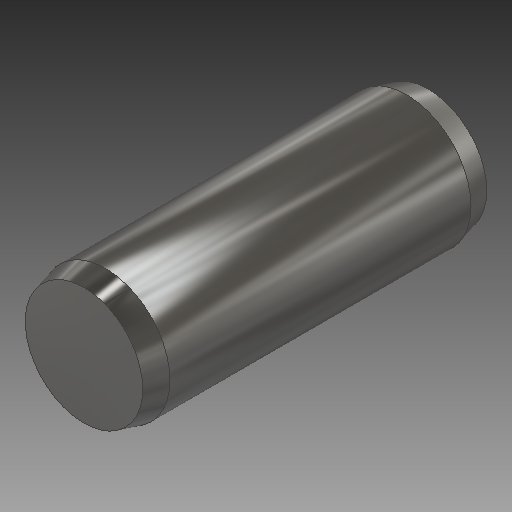
# Autodesk Inventor part: 平行ピンΦ3.8
Saved by Autodesk Inventor 2019 (Build 230136000, 136)
## iProperties
Created: 2018-07-18
Part Number: 平行ピンΦ3.8
Material: 鋼、高強度、低合金
Document SubType Name: Modeling
Designer: 雪村
Density: 7.85 g/cm^3
Appearance: 鋼 - つや出し
Mass: 0.439098 g
Surface Area: 0.870191 cm^2
Volume: 0.055936 cm^3
Author: 雪村
Autodesk Inventor part; units mm, degrees
ref_plane "YZ Plane" through (0, 0, 0) normal (1, 0, 0) x (0, 1, 0)
ref_plane "XZ Plane" through (0, 0, 0) normal (0, 1, 0) x (-1, 0, 0)
ref_plane "XY Plane" through (0, 0, 0) normal (0, 0, 1) x (1, 0, 0)
sketch "スケッチ1" plane through (0, 0, 0) normal (0, 0, 1) x (1, 0, 0)
  circle A0 centre (0, 0) radius 1.5
  dimension "d0" = 3
  constraints: 1 centre point, 1 coincident
  measures "d0" diameter of A0
extrude "押し出し1" add sketch "スケッチ1" along normal blind 8
chamfer "面取り1" distance 0.134 distance2 0.5 1 edges at (-1.5, 0, 8) measured on face at (0.3743, -0.3316, 8)
chamfer "面取り2" distance 0.134 distance2 0.5 1 edges at (-1.5, 0, 0) measured on face at (0.3743, -0.3316, 0)
